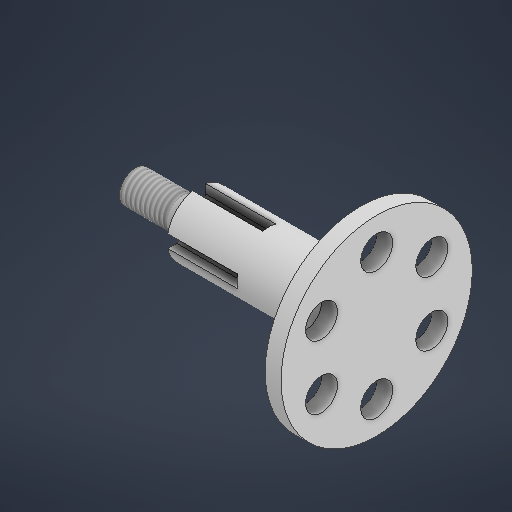
# Autodesk Inventor part: Hub-CV Adapter
Saved by Autodesk Inventor 2026.1 (Build 301233000, 233)
## iProperties
Created: 2026-06-12
Part Number: Hub-CV Adapter
Material: Generic
Document SubType Name: Modeling
Designer: share
Density: 1 g/cm^3
Appearance: Default
Author: share
Autodesk Inventor part; units mm, degrees
ref_plane "YZ Plane" through (0, 0, 0) normal (1, 0, 0) x (0, 1, 0)
ref_plane "XZ Plane" through (0, 0, 0) normal (0, 1, 0) x (-1, 0, 0)
sketch "Sketch1" plane through (0, 0, 0) normal (1, 0, 0) x (0, 1, 0)
  circle A0 centre (0, 0) radius 6.19 construction
  circle A1 centre (0, 0) radius 10
  dimension "d0" = 20
  dimension "d1" = 3.81
  constraints: 2 centre point, 2 coincident
  measures "d0" diameter of A1
  measures "d1" radial gap between concentric circles of A1 A0
extrude "Main Shaft" add sketch "Sketch1" against normal blind 50.8
sketch "Sketch2" plane through (0, 0, 0) normal (1, 0, 0) x (0, 0, -1)
  circle A0 centre (0, 0) radius 30
  dimension "d4" = 60
  constraints: 1 centre point, 1 coincident
  measures "d4" diameter of A0
extrude "CV Flange" add sketch "Sketch2" along normal blind 5
sketch "Sketch3" plane through (5, 0, 0) normal (1, 0, 0) x (0, 0, -1)
  circle A0 centre (0, 20) radius 5
  circle A1 centre (0, 0) radius 20 construction
  line L0 (0, 0) -> (0, 20) construction
  dimension "d7" = 40
  dimension "d8" = 10
  constraints: 2 end point, 1 centre point, 1 coincident, 1 vertical, 1 vertical alignment, 2 other
  measures "d8" diameter of A0
extrude "CV Bolt Hole" cut sketch "Sketch3" against normal up to surface (5 mm away)
pattern_circular "CV Bolt Pattern" count 6 over 360 about axis through (-10, 0, 0) along (1, 0, 0) of "CV Bolt Hole"
chamfer "Weld_Chamfer" distance 2 angle 45 1 edges at (0, -10, 0)
ref_plane "Lock Pin Hole Plane" through (0, 0, 12.7) normal (0, 0, 1) x (1, 0, 0)
sketch "Sketch5" plane through (-50.8, 0, 0) normal (-1, 0, 0) x (0, 0, 1)
  line L0 (-20, 0) -> (15, 0) construction
  line L1 (0, 14) -> (0, -14) construction
  arc A0 (-13, 2) -> (-13, -2) centre (-13, 0) ccw
  arc A1 (-7, -2) -> (-7, 2) centre (-7, 0) ccw
  line L2 (-13, -2) -> (-7, -2)
  line L3 (-13, 2) -> (-7, 2)
  point P0 (0, 0)
  dimension "d23" = 2
  dimension "d24" = 7
  dimension "d25" = 6
  constraints: 4 end point, 4 point on circle, 3 tangent, 2 centre point, 2 point on line, 1 equal radius, 1 horizontal
  measures "d23" radius of A0
  measures "d24" distance from line of L1 A1.centre
  measures "d25" distance of A1.centre A0.centre
extrude "Key Slot" cut sketch "Sketch5" against normal blind 22
pattern_circular "Circular Pattern2" count 4 over 360 about axis through (-10, 0, 0) along (1, 0, 0) of "Key Slot"
sketch "Sketch6" plane through (-50.8, 0, 0) normal (-1, 0, 0) x (0, 0, 1)
  circle A0 centre (0, 0) radius 5
  arc A1 (-7, -2) -> (-7, 2) centre (-7, 0) ccw projected
  constraints: 1 centre point, 1 coincident, 1 tangent
extrude "Extrusion6" add sketch "Sketch6" along normal blind 20
thread "M10x1.5 thread" size "M10x1.5" class "6g" standard "ANSI Metric M Profile" length 20 offset 5
equation "\"d1\" = Shaft_Wall_Thickness"
equation "\"d2\" = Shaft_Length"
equation "\"d4\" = Driveshaft_Flange_Diameter"
equation "\"d5\" = Driveshaft_Flange_Thickness"
equation "\"d7\" = CV_Bolt_Pattern_Diameter"
equation "\"d8\" = CV_Bolt_Hole_Diameter"
equation "\"Shaft_Diameter\" = 25.4"
equation "\"Shaft_Wall_Thickness\" = 3.81"
equation "\"Driveshaft_Flange_Diameter\" = 60"
equation "\"Driveshaft_Flange_Thickness\" = 5"
equation "\"CV_Bolt_Hole_Diameter\" = 10"
equation "\"d18\" = 0.5 * Shaft_Diameter"
equation "\"Shaft_Length\" = 50.8"
equation "\"CV_Bolt_Pattern_Diameter\" = 40"
body "Solid1"
